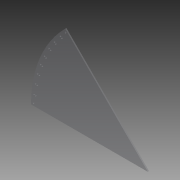
# Autodesk Inventor part: Side Panel
Saved by Autodesk Inventor 2013 (Build 170138000, 138)
## iProperties
Created: 2013-01-27
Part Number: Side Panel
Material: Polycarbonate, Clear
Document SubType Name: Modeling
Designer: Andrew Toennies
Density: 1.2 g/cm^3
Mass: 144.309 g
Surface Area: 790.745 cm^2
Volume: 120.258 cm^3
Author: Andrew Toennies
Autodesk Inventor part; units mm, degrees
ref_plane "YZ Plane" through (0, 0, 0) normal (1, 0, 0) x (0, 1, 0)
ref_plane "XZ Plane" through (0, 0, 0) normal (0, 1, 0) x (-1, 0, 0)
ref_plane "XY Plane" through (0, 0, 0) normal (0, 0, 1) x (1, 0, 0)
sketch "Sketch1" plane through (0, 0, 0) normal (0, 0, 1) x (1, 0, 0)
  arc A0 (-220.0163, 220.0163) -> (-311.15, 0) centre (0, 0) ccw
  line L0 (-311.15, 0) -> (-304.8, 0)
  line L1 (0, 0) -> (-220.0163, 220.0163)
  line L2 (-311.15, 0) -> (0, 0)
  constraints: 6 end point, 2 point on circle, 1 centre point
extrude "Extrusion1" add sketch "Sketch1" along normal blind 3.175
sketch "Sketch4" plane through (0, 0, 0) normal (0, 0, -1) x (-1, 0, 0)
  arc A0 (311.15, 0) -> (220.0163, 220.0163) centre (0, 0) ccw projected
  line L0 (220.0163, 220.0163) -> (0, 0) projected
  line L1 (0, 0) -> (311.15, 0) projected
  arc A1 (301.625, 0) -> (213.2811, 213.2811) centre (0, 0) ccw
  arc A2 (303.2125, 0) -> (214.4036, 214.4036) centre (0, 0) ccw
  arc A3 (304.8, 0) -> (215.5261, 215.5261) centre (0, 0) ccw construction
  arc A4 (300.0375, 0) -> (212.1586, 212.1586) centre (0, 0) ccw construction
  circle A5 centre (215.5261, 215.5261) radius 1.5875
  circle A6 centre (212.1586, 212.1586) radius 1.5875
  circle A7 centre (233.4903, 195.9217) radius 1.5875
  circle A8 centre (229.8421, 192.8604) radius 1.5875
  circle A9 centre (249.6775, 174.8261) radius 1.5875
  circle A10 centre (245.7763, 172.0944) radius 1.5875
  circle A11 centre (263.9645, 152.4) radius 1.5875
  circle A12 centre (259.8401, 150.0188) radius 1.5875
  circle A13 centre (276.2426, 128.814) radius 1.5875
  circle A14 centre (271.9263, 126.8013) radius 1.5875
  circle A15 centre (286.4183, 104.2477) radius 1.5875
  circle A16 centre (281.943, 102.6189) radius 1.5875
  circle A17 centre (294.4142, 78.888) radius 1.5875
  circle A18 centre (289.814, 77.6554) radius 1.5875
  circle A19 centre (300.1694, 52.928) radius 1.5875
  circle A20 centre (295.4793, 52.101) radius 1.5875
  circle A21 centre (303.6401, 26.5651) radius 1.5875
  circle A22 centre (298.8958, 26.15) radius 1.5875
  circle A23 centre (304.8, 0) radius 1.5875
  circle A24 centre (300.0375, 0) radius 1.5875
  circle A25 centre (219.9695, 210.9892) radius 1.5875
  circle A26 centre (304.7338, 6.35) radius 1.5875
  point P0 (231.0582, 193.8808)
  point P1 (232.2743, 194.9012)
  point P2 (247.0767, 173.005)
  point P3 (248.3771, 173.9155)
  point P4 (261.2149, 150.8125)
  point P5 (262.5897, 151.6063)
  point P6 (273.3651, 127.4722)
  point P7 (274.8038, 128.1431)
  point P8 (283.4348, 103.1618)
  point P9 (284.9265, 103.7048)
  point P10 (291.3474, 78.0663)
  point P11 (292.8808, 78.4772)
  point P12 (297.0426, 52.3766)
  point P13 (298.606, 52.6523)
  point P14 (300.4772, 26.2884)
  point P15 (302.0587, 26.4267)
  point P16 (301.625, 0)
  point P17 (303.2125, 0)
  dimension "d2" = 9.525
  dimension "d3" = 1.5875
  dimension "d4" = 1.5875
  dimension "d5" = 1.5875
  dimension "d8" = 45
  dimension "d10" = 6.35
  dimension "d13" = 3.175
  dimension "d14" = 6.35
  constraints: 10 point on circle, 6 centre point, 2 coincident, 2 horizontal alignment, 2 point on line, 1 tangent, 113 other
  measures "d2" radial gap between concentric circles of A0 A1
  measures "d3" radial gap between concentric circles of A2 A1
  measures "d4" radial gap between concentric circles of A4 A1
  measures "d5" radial gap between concentric circles of A3 A2
  measures "d10" distance from line of L0 A25.centre
  measures "d13" diameter of A26
  measures "d14" distance from line of L1 A26.centre
extrude "Extrusion2" cut sketch "Sketch4" against normal blind 25.4 contours A25 | A7 | A9 | A11 | A13 | A15 | A17 | A19 | A21 | A26 | A22 | A20 | A18 | A16 | A14 | A12 | A10 | A8
body "Solid1"
